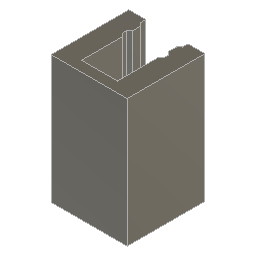
Крепление пневматического инструмента_ver2 (Autodesk Fusion 360 design; units mm, degrees)
Autodesk Fusion 360 part; units mm, degrees
sketch "Sketch1" plane through (0, 0, 0) normal (0, 0, 1) x (1, 0, 0)
  line L0 (5.2, 0.9172) -> (5.2, -11)
  line L1 (6.1, 1.8172) -> (5.2, 0.9172)
  line L2 (6.1, 2.8828) -> (6.1, 1.8172)
  line L3 (5.2, 3.7828) -> (6.1, 2.8828)
  line L4 (5.2, 6.1172) -> (5.2, 3.7828)
  line L5 (6.1, 7.0172) -> (5.2, 6.1172)
  line L6 (6.1, 8.5) -> (6.1, 7.0172)
  line L7 (6.1, 8.5) -> (7, 8.5)
  line L8 (7, 8.5) -> (11, 8.5)
  line L9 (11, 8.5) -> (11, -14)
  line L10 (11, -14) -> (0, -14)
  line L11 (0, -11) -> (5.2, -11)
  arc A0 (0, -8.75) -> (0, -5.25) centre (0, -7) ccw
  arc A1 (0, 2.25) -> (0, 5.75) centre (0, 4) ccw
  line L12 (0, 1.75) -> (0, 22.5)
  arc A2 (0, 5.75) -> (0, 2.25) centre (0, 4) ccw
  line L13 (-6.1, 8.5) -> (-6.1, 7.0172)
  line L14 (-6.1, 8.5) -> (-7, 8.5)
  line L15 (-7, 8.5) -> (-11, 8.5)
  line L16 (-6.1, 2.8828) -> (-6.1, 1.8172)
  line L17 (-11, -14) -> (0, -14)
  line L18 (-11, 8.5) -> (-11, -14)
  arc A3 (0, -5.25) -> (0, -8.75) centre (0, -7) ccw
  line L19 (-6.1, 1.8172) -> (-5.2, 0.9172)
  line L20 (-6.1, 7.0172) -> (-5.2, 6.1172)
  line L21 (0, -11) -> (-5.2, -11)
  line L22 (-5.2, 0.9172) -> (-5.2, -11)
  line L23 (-5.2, 3.7828) -> (-6.1, 2.8828)
  line L24 (-5.2, 6.1172) -> (-5.2, 3.7828)
  line L25 (6.1, 8.5) -> (-6.1, 8.5)
  dimension "d1" = 3.5
  dimension "d2" = 3.5
  constraint perpendicular L6 L7
  constraint perpendicular L6 L8
  constraint perpendicular L8 L9
  constraint perpendicular L9 L10
  constraint horizontal L11
  constraint symmetric L6.start L12 L13.start
  constraint symmetric L1.start L12 L16.end
  constraint symmetric L5.start L12 L13.end
  constraint symmetric L3.start L12 L23.start
  constraint symmetric L2.start L12 L16.start
  constraint symmetric L4.start L12 L20.end
  constraint symmetric L0.start L12 L19.end
  constraint symmetric L7.end L12 L14.end
  constraint symmetric L8.end L12 L15.end
  constraint symmetric L9.end L12 L17.start
  constraint symmetric L10.end L12 L17.end
  constraint symmetric L11.start L12 L21.start
  constraint symmetric L0.end L12 L21.end
  constraint symmetric A0.end L12 A3.start
  constraint symmetric A0.start L12 A3.end
  constraint symmetric A0 L12 A3
  constraint symmetric A1.end L12 A2.start
  constraint symmetric A1.start L12 A2.end
  constraint symmetric A1 L12 A2
  measures "d1" diameter of A0
  measures "d2" diameter of A1
extrude "Extrude1" add sketch "Sketch1" along normal blind 3
extrude "Extrude2" add sketch "Sketch1" along normal blind 37 contours L0 L1 L2 L3 L4 L5 L6 L7 L8 L9 L10 L11 L13 L14 L15 L16 L17 L18 L19 L20 L21 L22 L23 L24
chamfer "Chamfer1" distance 1 angle 45 2 edges at (-0.6328, 2.3684, 3) (-0.6328, -8.6316, 3)
